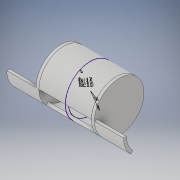
# Autodesk Inventor part: custom support at hinge V2
Saved by Autodesk Inventor 2019 (Build 230136000, 136)
## iProperties
Created: 2018-07-06
Part Number: custom support at hinge V2
Material: Generic
Document SubType Name: Modeling
Designer: HIVE
Density: 1 g/cm^3
Appearance: Default
Author: HIVE
Autodesk Inventor part; units mm, degrees
ref_plane "YZ Plane" through (0, 0, 0) normal (1, 0, 0) x (0, 1, 0)
ref_plane "XZ Plane" through (0, 0, 0) normal (0, 1, 0) x (-1, 0, 0)
ref_plane "XY Plane" through (0, 0, 0) normal (0, 0, 1) x (1, 0, 0)
sketch "Sketch3" plane through (0, 0, 0) normal (1, 0, 0) x (0, 1, 0)
  circle A0 centre (0, 0) radius 5.5
  circle A1 centre (0, 0) radius 7.5
  circle A2 centre (0, 0) radius 8.5
  circle A3 centre (0, 0) radius 5
  line L0 (-5.3033, 5.3033) -> (-6.0104, 6.0104)
  line L1 (0, 7.5) -> (0, 8.5)
  dimension "d45" = 11
  dimension "d46" = 15
  dimension "d47" = 17
  dimension "d52" = 10
  constraints: 4 centre point, 4 coincident, 4 end point, 4 point on circle, 1 vertical
  measures "d45" diameter of A0
  measures "d46" diameter of A1
  measures "d47" diameter of A2
  measures "d52" diameter of A3
extrude "Extrusion14" add sketch "Sketch3" along normal mid plane 18 contours A0 | A1 L1 A2 L0 picked at (-7.7922, -2.2519)
extrude "Extrusion13" add sketch "Sketch3" along normal blind 1 from surface at 9 separate body contours A0 | A1 | A1 L1 A2 L0 | A1 L0 A2 L1 | A3
extrude "Extrusion15" add sketch "Sketch3" along normal blind 10 from surface at 10 separate body contours A1 L0 A2 L1 picked at (-2.1248, 7.8485)
mirror "Mirror1" about plane through (0, 0, 0) normal (1, 0, 0) of "Extrusion13", "Extrusion15" bodies 2
equation "\"d45\" = circle1"
equation "\"d46\" = circle2"
equation "\"d47\" = circle3"
equation "\"d52\" = circle0"
equation "\"d54\" = distance0"
equation "\"d50\" = clearance"
equation "\"distance0\" = 0.5 * legDiam - 2 * clearance"
equation "\"circle1\" = kneeBallBaseH + clearance"
equation "\"circle0\" = kneeBallBaseH"
equation "\"distance1\" = 1"
equation "\"circle2\" = 15"
equation "\"circle3\" = 17"
equation "\"clearance\" = 1"
equation "\"legDiam\" = 40"
equation "\"kneeBallBaseH\" = 10"
body "Solid2"
body "Solid3"
body "Solid4"
